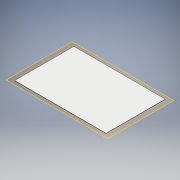
# Autodesk Inventor part: BusinessCard
Saved by Autodesk Inventor 2017 (Build 210142000, 142)
## iProperties
Created: 2017-09-13
Part Number: BusinessCard
Material: Rubber
Document SubType Name: Modeling
Designer: erwin
Density: 0.93 g/cm^3
Appearance: White
Author: erwin
Autodesk Inventor part; units mm, degrees
ref_plane "YZ Plane" through (0, 0, 0) normal (1, 0, 0) x (0, 1, 0)
ref_plane "XZ Plane" through (0, 0, 0) normal (0, 1, 0) x (-1, 0, 0)
ref_plane "XY Plane" through (0, 0, 0) normal (0, 0, 1) x (1, 0, 0)
ref_plane "Work Plane1" through (0, 0, 0) normal (0, 0, 1) x (1, 0, 0)
sketch "Sketch1" plane through (0, 0, 0) normal (0, 0, 1) x (1, 0, 0)
  line L0 (-42.604, -15.0136) -> (43.396, -15.0136) construction
  line L1 (-42.604, -15.0136) -> (43.396, -15.0136) construction
  line L2 (0.396, 12.9864) -> (0.396, -43.0136) construction
  line L3 (-42.104, -42.5136) -> (42.896, -42.5136)
  line L4 (42.896, -42.5136) -> (42.896, 12.4864)
  line L5 (42.896, 12.4864) -> (-42.104, 12.4864)
  line L6 (-42.104, 12.4864) -> (-42.104, -42.5136)
  line L7 (-42.104, -42.5136) -> (42.896, 12.4864) construction
  line L8 (42.896, -42.5136) -> (-42.104, 12.4864) construction
  point P0 (0.396, -15.0136)
  dimension "d3" = 85
  dimension "d4" = 55
  constraints: 18 end point, 3 midpoint, 2 horizontal, 2 parallel, 1 collinear, 1 perpendicular, 1 vertical
  measures "d3" distance of L5.end L4.end
  measures "d4" distance of L4.end L3.end
extrude "Extrusion1" add sketch "Sketch1" along normal blind 0.3
body "Solid1"
